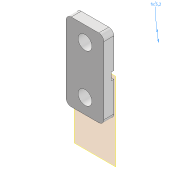
# Autodesk Inventor part: tampa_suporte_termopar
Saved by Autodesk Inventor 2020 (Build 240168000, 168)
## iProperties
Created: 2022-07-21
Part Number: tampa_suporte_termopar
Material: Genérico
Document SubType Name: Modeling
Designer: gabri
Density: 1 g/cm^3
Appearance: Padrão
Author: gabri
Autodesk Inventor part; units mm, degrees
ref_plane "YZ Plane" through (0, 0, 0) normal (1, 0, 0) x (0, 1, 0)
ref_plane "XZ Plane" through (0, 0, 0) normal (0, 1, 0) x (-1, 0, 0)
ref_plane "XY Plane" through (0, 0, 0) normal (0, 0, 1) x (1, 0, 0)
ref_plane "Plano de trabalho1" through (0, 0, 0) normal (0, 0, 1) x (1, 0, 0)
sketch "Esboço1" plane through (0, 0, 0) normal (0, 0, 1) x (1, 0, 0)
  circle A0 centre (0, 9.5) radius 2.6
  line L0 (-7.5, -1.5) -> (-7.5, 1.5)
  line L1 (7.5, -1.5) -> (-7.5, -1.5)
  line L2 (7.5, 1.5) -> (7.5, -1.5)
  line L3 (-7.5, 1.5) -> (7.5, 1.5)
  circle A1 centre (0, -9.5) radius 2.6
  line L4 (-7.5, 1.5) -> (7.5, 1.5)
  line L5 (7.5, 1.5) -> (7.5, 15.5)
  line L6 (-7.5, 15.5) -> (-7.5, 1.5)
  circle A2 centre (0, 9.5) radius 2.1
  line L7 (7.5, -1.5) -> (-7.5, -1.5)
  line L8 (-7.5, -1.5) -> (-7.5, -15.5)
  line L9 (7.5, -15.5) -> (7.5, -1.5)
  circle A3 centre (0, -9.5) radius 2.1
  line L10 (-7.5, 15.5) -> (7.5, 15.5)
  line L11 (7.5, 15.5) -> (7.5, -15.5)
  line L12 (7.5, -15.5) -> (-7.5, -15.5)
  line L13 (-7.5, -15.5) -> (-7.5, 15.5)
  point P0 (0, 0)
  dimension "d0" = 14
  dimension "d1" = 14
  dimension "d7" = 5.2
  dimension "d8" = 5.2
  constraints: 28 end point, 4 centre point
  measures "d0" distance between parallel lines of L3 L10
  measures "d1" distance between parallel lines of L12 L1
  measures "d7" diameter of A0
  measures "d8" diameter of A1
extrude "Extrusão1" add sketch "Esboço1" along normal blind 4 contours L0 L3 L2 L1 | L1 L9 L12 L8 | L6 L10 L5 L3
extrude "Extrusão2" cut sketch "Esboço1" along normal blind 1 contours L0 L3 L2 L1
fillet "Arredondamento1" radius 2 4 edges at (-7.5, 15.5, 2) (7.5, 15.5, 2) (-7.5, -15.5, 2) (7.5, -15.5, 2)
equation "\"d1\" = d0"
equation "\"d8\" = d7"
